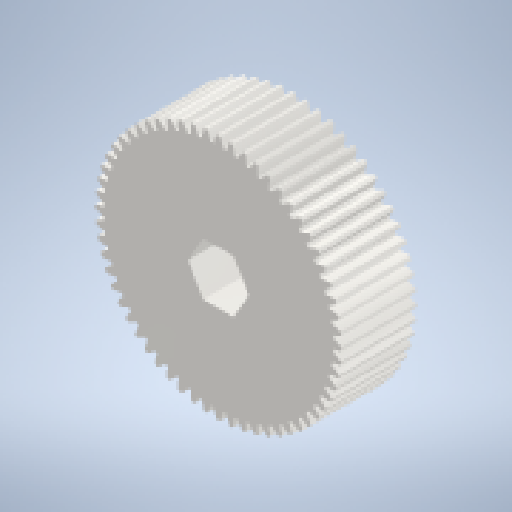
# Autodesk Inventor part: Spur Gear2
Saved by Autodesk Inventor 2024 (Build 280153020, 153B)
## iProperties
Created: 2024-04-17
Part Number: Spur Gear2
Material: Steel
Document SubType Name: Modeling
Designer: lvrectanus0
Categories: <?xml version="1.0" encoding="UTF-16"?> <MemberInstance><Categories><FamilyTemplate><FamilyTemplateParameter ValueType="xs:double" Id="1" ObjectReferenceKey="da_z" ObjectType="kUserParameterObject"/><FamilyTemplateParameter ValueType="xs:double" Id="2" ObjectReferenceKey="da_b" ObjectType="kUserParameterObject"/><FamilyTemplateParameter ValueType="xs:double" Id="3" ObjectReferenceKey="da_beta" ObjectType="kUserParameterObject"/><FamilyTemplateParameter ValueType="xs:double" Id="4" ObjectReferenceKey="da_da" ObjectType="kUserParameterObject"/><FamilyTemplateParameter ValueType="xs:double" Id="5" ObjectReferenceKey="da_aw" ObjectType="kUserParameterObject"/><FamilyTemplateParameter ValueType="xs:string" Id="6" ObjectReferenceKey="EAIAABAAAAC/AAAAAAAAAIAAAAAAAAAA" ObjectType="83910656" SubObjectId="SurfaceGeometry"/></FamilyTemplate><ParamToTemplateMap><ParamToTemplate CategoryParameter="//CategoryParameter[@InternalName='046C89C9-8512-4d59-83FE-43B91F4F132A']" TemplateParameter="1"/><ParamToTemplate CategoryParameter="//CategoryParameter[@InternalName='2552DF32-E462-4b46-AEBF-C6C7768E72AC']" TemplateParameter="2"/><ParamToTemplate CategoryParameter="//CategoryParameter[@InternalName='C9EE641D-15FC-4fae-A226-E94C4372FDD7']" TemplateParameter="3"/><ParamToTemplate><ParamToTemplate CategoryParameter="//CategoryParameter[@InternalName='00B6519A-459B-49c7-AD84-2E56D39A5744']" ConstantValue="0.000000"/></ParamToTemplate><ParamToTemplate><ParamToTemplate CategoryParameter="//CategoryParameter[@InternalName='04B31F0E-C7A6-4894-AA32-9629BEFACF47']" ConstantValue="1.000000"/></ParamToTemplate><ParamToTemplate><ParamToTemplate CategoryParameter="//CategoryParameter[@InternalName='43CBEC2E-7847-49e7-A936-2F7889FCB2D9']" ConstantValue="0.250000"/></ParamToTemplate><ParamToTemplate><ParamToTemplate CategoryParameter="//CategoryParameter[@InternalName='B1EFC894-105D-4ebd-86BF-FA20ED196853']" ConstantValue="0.350000"/></ParamToTemplate><ParamToTemplate><ParamToTemplate CategoryParameter="//CategoryParameter[@InternalName='51175063-3D10-4879-93E8-6246FE8B403D']" ConstantValue="2061532430.657340"/></ParamToTemplate><ParamToTemplate><ParamToTemplate CategoryParameter="//CategoryParameter[@InternalName='A3A52E27-4454-46a9-B0BD-C932399B70AF']" ConstantValue="0.300000"/></ParamToTemplate><ParamToTemplate><ParamToTemplate CategoryParameter="//CategoryParameter[@InternalName='91B76062-C214-41d9-B1B9-14D2AB99603D']" ConstantValue="0.079375"/></ParamToTemplate><ParamToTemplate><ParamToTemplate CategoryParameter="//CategoryParameter[@InternalName='374E806E-8B8A-4dda-A9AA-1039D6500AD2']" ConstantValue="12.598425"/></ParamToTemplate><ParamToTemplate><ParamToTemplate CategoryParameter="//CategoryParameter[@InternalName='2D373A89-B862-43d6-8D0B-0CBF12AB9F6C']" ConstantValue="0.349066"/></ParamToTemplate><ParamToTemplate CategoryParameter="//CategoryParameter[@InternalName='37777632-D6A2-4fac-9D53-DB8ACD95C989']" TemplateParameter="4"/><ParamToTemplate CategoryParameter="//CategoryParameter[@InternalName='FD1017F1-B727-4f7e-9707-0F86F1FF9423']" TemplateParameter="5"/><ParamToTemplate><ParamToTemplate CategoryParameter="//CategoryParameter[@InternalName='9E1B4470-B2D3-4ff1-B813-535BB4CDF51A']" ConstantValue="3523220.976809"/></ParamToTemplate><ParamToTemplate><ParamToTemplate CategoryParameter="//CategoryParameter[@InternalName='F8452263-BFF6-458c-9FB1-07C4B99E95CD']" ConstantValue="11397033.805607"/></ParamToTemplate><ParamToTemplate><ParamToTemplate CategoryParameter="//CategoryParameter[@InternalName='3E3BB259-FD49-497f-8171-6EBC954A3479']" ConstantValue="2.000000"/></ParamToTemplate><ParamToTemplate CategoryParameter="//CategoryParameter[@InternalName='27C3BAF2-7550-4e4b-AE2C-0DB134B7D9B7']" TemplateParameter="6"/></ParamToTemplateMap><Category DisplayName="Gear" InternalName="DC85795E-93AB-48d5-8EEE-5A27447B64BD" Mnemonic="Gear"><CategoryParameter DisplayName="z" InternalName="046C89C9-8512-4d59-83FE-43B91F4F132A" Mnemonic="z"/><CategoryParameter DisplayName="b" InternalName="2552DF32-E462-4b46-AEBF-C6C7768E72AC" Mnemonic="b"/><CategoryParameter DisplayName="||b|" InternalName="C9EE641D-15FC-4fae-A226-E94C4372FDD7" Mnemonic="beta"/><CategoryParameter DisplayName="x" InternalName="00B6519A-459B-49c7-AD84-2E56D39A5744" Mnemonic="x"/><CategoryParameter DisplayName="a*" InternalName="04B31F0E-C7A6-4894-AA32-9629BEFACF47" Mnemonic="a"/><CategoryParameter DisplayName="c*" InternalName="43CBEC2E-7847-49e7-A936-2F7889FCB2D9" Mnemonic="c"/><CategoryParameter DisplayName="r|.f|*" InternalName="B1EFC894-105D-4ebd-86BF-FA20ED196853" Mnemonic="rf"/><CategoryParameter DisplayName="E" InternalName="51175063-3D10-4879-93E8-6246FE8B403D" Mnemonic="E"/><CategoryParameter DisplayName="||m|" InternalName="A3A52E27-4454-46a9-B0BD-C932399B70AF" Mnemonic="mi"/><Category DisplayName="SpurGear" InternalName="26C5A22E-A91E-4dfd-A3B3-23CCAFAE1764" Mnemonic="SpurGear"><CategoryParameter DisplayName="m" InternalName="91B76062-C214-41d9-B1B9-14D2AB99603D" Mnemonic="m"/><CategoryParameter DisplayName="P" InternalName="374E806E-8B8A-4dda-A9AA-1039D6500AD2" Mnemonic="PP"/><CategoryParameter DisplayName="||a|" InternalName="2D373A89-B862-43d6-8D0B-0CBF12AB9F6C" Mnemonic="alpha"/><CategoryParameter DisplayName="d|.a|" InternalName="37777632-D6A2-4fac-9D53-DB8ACD95C989" Mnemonic="da"/><CategoryParameter DisplayName="a|.w|" InternalName="FD1017F1-B727-4f7e-9707-0F86F1FF9423" Mnemonic="aw"/><CategoryParameter DisplayName="||s||.Flim|" InternalName="9E1B4470-B2D3-4ff1-B813-535BB4CDF51A" Mnemonic="sFlim"/><CategoryParameter DisplayName="||s||.Hlim|" InternalName="F8452263-BFF6-458c-9FB1-07C4B99E95CD" Mnemonic="sHlim"/><CategoryParameter DisplayName="type" InternalName="3E3BB259-FD49-497f-8171-6EBC954A3479" Mnemonic="type"/><CategoryParameter DisplayName="PitchDiameter" InternalName="27C3BAF2-7550-4e4b-AE2C-0DB134B7D9B7" Mnemonic="IDS_PITCHDIAM"/></Category></Category></Categories></MemberInstance>
Density: 1 g/cm^3
Appearance: Steel
CustomPartVersion: 1
Author: lvrectanus0
Autodesk Inventor part; units mm, degrees
ref_plane "YZ Plane" through (0, 0, 0) normal (1, 0, 0) x (0, 1, 0)
ref_plane "XZ Plane" through (0, 0, 0) normal (0, 1, 0) x (-1, 0, 0)
ref_plane "XY Plane" through (0, 0, 0) normal (0, 0, 1) x (1, 0, 0)
sketch "Sketch1" plane through (0, 0, 0) normal (0, 0, 1) x (1, 0, 0)
  circle A0 centre (0, 0) radius 24.6062
  dimension "d0" = 49.2125
  constraints: 1 centre point
  measures "d0" diameter of A0
extrude "Extrusion1" add sketch "Sketch1" along normal blind 15
sketch "Sketch2" plane through (0, 0, 0) normal (0, 0, -1) x (-1, 0, 0)
  circle A0 centre (0, 0) radius 24.6062 projected
  circle A1 centre (0, 0) radius 23.8125
  dimension "d3" = 47.625
  constraints: 1 centre point, 1 coincident
  measures "d3" diameter of A1
surface extrude "Pitch Diameter" sketch "Sketch2" against normal through all shown no curves A1
ref_plane "Work Plane1" through (0, 0, 0) normal (1, 0, 0) x (0, 1, 0)
ref_plane "Work Plane2" through (0, 0, 0) normal (0.9986295, 0.052336, 0) x (0, 0, 1)
ref_plane "Work Plane3" through (0, 0, 7.5) normal (0, 0, -1) x (-1, 0, 0)
spur gear teeth "Spur Gear" teeth 60 pitch diameter 47.625 tip diameter 49.2125 root diameter 45.6406 face width 50.8 start plane through (0, 0, 0) normal (0, 0, -1) x (-1, 0, 0)
sketch "Sketch3" plane through (0, 0, 15) normal (0, 0, 1) x (1, 0, 0)
  line L0 (-3.0383, 5.2625) -> (3.0383, 5.2625)
  line L1 (3.0383, 5.2625) -> (6.0766, 0)
  line L2 (6.0766, 0) -> (3.0383, -5.2625)
  line L3 (3.0383, -5.2625) -> (-3.0383, -5.2625)
  line L4 (-3.0383, -5.2625) -> (-6.0766, 0)
  line L5 (-6.0766, 0) -> (-3.0383, 5.2625)
  line L6 (-3.0383, 5.2625) -> (3.0383, -5.2625)
  line L7 (-6.0766, 0) -> (6.0766, 0)
  line L8 (3.0383, 5.2625) -> (-3.0383, -5.2625)
  arc A0 (-2.8922, 24.4357) -> (-3.2745, 22.5842) centre (6.6821, 21.4931) ccw projected
  arc A1 (-3.2745, 22.5842) -> (-3.8646, 22.4907) centre (0, 0) ccw projected
  arc A2 (-3.8646, 22.4907) -> (-4.8004, 24.1334) centre (-12.9968, 18.3763) ccw projected
  arc A3 (-4.8004, 24.1334) -> (-5.4305, 23.9995) centre (0, 0) ccw projected
  arc A4 (-5.4305, 23.9995) -> (-5.6173, 22.1182) centre (4.3989, 22.0738) ccw projected
  arc A5 (-5.6173, 22.1182) -> (-6.1944, 21.9635) centre (0, 0) ccw projected
  arc A6 (-6.1944, 21.9635) -> (-7.2968, 23.4995) centre (-14.8464, 16.9171) ccw projected
  arc A7 (-7.2968, 23.4995) -> (-7.9094, 23.3004) centre (0, 0) ccw projected
  arc A8 (-7.9094, 23.3004) -> (-7.8985, 21.4098) centre (2.0674, 22.4127) ccw projected
  arc A9 (-7.8985, 21.4098) -> (-8.4562, 21.1957) centre (0, 0) ccw projected
  arc A10 (-8.4562, 21.1957) -> (-9.7132, 22.608) centre (-16.5334, 15.2725) ccw projected
  arc A11 (-9.7132, 22.608) -> (-10.3016, 22.346) centre (0, 0) ccw projected
  arc A12 (-10.3016, 22.346) -> (-10.0932, 20.4669) centre (-0.2867, 22.506) ccw projected
  arc A13 (-10.0932, 20.4669) -> (-10.6255, 20.1957) centre (0, 0) ccw projected
  arc A14 (-10.6255, 20.1957) -> (-12.0231, 21.4689) centre (-18.0393, 13.4606) ccw projected
  arc A15 (-12.0231, 21.4689) -> (-12.581, 21.1468) centre (0, 0) ccw projected
  arc A16 (-12.581, 21.1468) -> (-12.1773, 19.2998) centre (-2.6376, 22.3528) ccw projected
  arc A17 (-12.1773, 19.2998) -> (-12.6783, 18.9744) centre (0, 0) ccw projected
  arc A18 (-12.6783, 18.9744) -> (-14.2014, 20.0945) centre (-19.3475, 11.5013) ccw projected
  arc A19 (-14.2014, 20.0945) -> (-14.7225, 19.7159) centre (0, 0) ccw projected
  arc A20 (-14.7225, 19.7159) -> (-14.1279, 17.9212) centre (-4.9597, 21.9546) ccw projected
  arc A21 (-14.1279, 17.9212) -> (-14.5922, 17.5452) centre (0, 0) ccw projected
  arc A22 (-14.5922, 17.5452) -> (-16.224, 18.5) centre (-20.4437, 9.4159) ccw projected
  arc A23 (-16.224, 18.5) -> (-16.7027, 18.0689) centre (0, 0) ccw projected
  arc A24 (-16.7027, 18.0689) -> (-15.9238, 16.3462) centre (-7.2274, 21.3159) ccw projected
  arc A25 (-15.9238, 16.3462) -> (-16.3462, 15.9238) centre (0, 0) ccw projected
  arc A26 (-16.3462, 15.9238) -> (-18.0689, 16.7027) centre (-21.3159, 7.2274) ccw projected
  arc A27 (-18.0689, 16.7027) -> (-18.5, 16.224) centre (0, 0) ccw projected
  arc A28 (-18.5, 16.224) -> (-17.5452, 14.5922) centre (-9.4159, 20.4437) ccw projected
  arc A29 (-17.5452, 14.5922) -> (-17.9212, 14.1279) centre (0, 0) ccw projected
  arc A30 (-17.9212, 14.1279) -> (-19.7159, 14.7225) centre (-21.9546, 4.9597) ccw projected
  arc A31 (-19.7159, 14.7225) -> (-20.0945, 14.2014) centre (0, 0) ccw projected
  arc A32 (-20.0945, 14.2014) -> (-18.9744, 12.6783) centre (-11.5013, 19.3475) ccw projected
  arc A33 (-18.9744, 12.6783) -> (-19.2998, 12.1773) centre (0, 0) ccw projected
  arc A34 (-19.2998, 12.1773) -> (-21.1468, 12.581) centre (-22.3528, 2.6376) ccw projected
  arc A35 (-21.1468, 12.581) -> (-21.4689, 12.0231) centre (0, 0) ccw projected
  arc A36 (-21.4689, 12.0231) -> (-20.1957, 10.6255) centre (-13.4606, 18.0393) ccw projected
  arc A37 (-20.1957, 10.6255) -> (-20.4669, 10.0932) centre (0, 0) ccw projected
  arc A38 (-20.4669, 10.0932) -> (-22.346, 10.3016) centre (-22.506, 0.2867) ccw projected
  arc A39 (-22.346, 10.3016) -> (-22.608, 9.7132) centre (0, 0) ccw projected
  arc A40 (-22.608, 9.7132) -> (-21.1957, 8.4562) centre (-15.2725, 16.5334) ccw projected
  arc A41 (-21.1957, 8.4562) -> (-21.4098, 7.8985) centre (0, 0) ccw projected
  arc A42 (-21.4098, 7.8985) -> (-23.3004, 7.9094) centre (-22.4127, -2.0674) ccw projected
  arc A43 (-23.3004, 7.9094) -> (-23.4995, 7.2968) centre (0, 0) ccw projected
  arc A44 (-23.4995, 7.2968) -> (-21.9635, 6.1944) centre (-16.9171, 14.8464) ccw projected
  arc A45 (-21.9635, 6.1944) -> (-22.1182, 5.6173) centre (0, 0) ccw projected
  arc A46 (-22.1182, 5.6173) -> (-23.9995, 5.4305) centre (-22.0738, -4.3989) ccw projected
  arc A47 (-23.9995, 5.4305) -> (-24.1334, 4.8004) centre (0, 0) ccw projected
  arc A48 (-24.1334, 4.8004) -> (-22.4907, 3.8646) centre (-18.3763, 12.9968) ccw projected
  arc A49 (-22.4907, 3.8646) -> (-22.5842, 3.2745) centre (0, 0) ccw projected
  arc A50 (-22.5842, 3.2745) -> (-24.4357, 2.8922) centre (-21.4931, -6.6821) ccw projected
  arc A51 (-24.4357, 2.8922) -> (-24.503, 2.2515) centre (0, 0) ccw projected
  arc A52 (-24.503, 2.2515) -> (-22.7715, 1.4925) centre (-19.6341, 11.0048) ccw projected
  arc A53 (-22.7715, 1.4925) -> (-22.8027, 0.8959) centre (0, 0) ccw projected
  arc A54 (-22.8027, 0.8959) -> (-24.6041, 0.3221) centre (-20.6769, -8.8921) ccw projected
  arc A55 (-24.6041, 0.3221) -> (-24.6041, -0.3221) centre (0, 0) ccw projected
  arc A56 (-24.6041, -0.3221) -> (-22.8027, -0.8959) centre (-20.6769, 8.8921) ccw projected
  arc A57 (-22.8027, -0.8959) -> (-22.7715, -1.4925) centre (0, 0) ccw projected
  arc A58 (-22.7715, -1.4925) -> (-24.503, -2.2515) centre (-19.6341, -11.0048) ccw projected
  arc A59 (-24.503, -2.2515) -> (-24.4357, -2.8922) centre (0, 0) ccw projected
  arc A60 (-24.4357, -2.8922) -> (-22.5842, -3.2745) centre (-21.4931, 6.6821) ccw projected
  arc A61 (-22.5842, -3.2745) -> (-22.4907, -3.8646) centre (0, 0) ccw projected
  arc A62 (-22.4907, -3.8646) -> (-24.1334, -4.8004) centre (-18.3763, -12.9968) ccw projected
  arc A63 (-24.1334, -4.8004) -> (-23.9995, -5.4305) centre (0, 0) ccw projected
  arc A64 (-23.9995, -5.4305) -> (-22.1182, -5.6173) centre (-22.0738, 4.3989) ccw projected
  arc A65 (-22.1182, -5.6173) -> (-21.9635, -6.1944) centre (0, 0) ccw projected
  arc A66 (-21.9635, -6.1944) -> (-23.4995, -7.2968) centre (-16.9171, -14.8464) ccw projected
  arc A67 (-23.4995, -7.2968) -> (-23.3004, -7.9094) centre (0, 0) ccw projected
  arc A68 (-23.3004, -7.9094) -> (-21.4098, -7.8985) centre (-22.4127, 2.0674) ccw projected
  arc A69 (-21.4098, -7.8985) -> (-21.1957, -8.4562) centre (0, 0) ccw projected
  arc A70 (-21.1957, -8.4562) -> (-22.608, -9.7132) centre (-15.2725, -16.5334) ccw projected
  arc A71 (-22.608, -9.7132) -> (-22.346, -10.3016) centre (0, 0) ccw projected
  arc A72 (-22.346, -10.3016) -> (-20.4669, -10.0932) centre (-22.506, -0.2867) ccw projected
  arc A73 (-20.4669, -10.0932) -> (-20.1957, -10.6255) centre (0, 0) ccw projected
  arc A74 (-20.1957, -10.6255) -> (-21.4689, -12.0231) centre (-13.4606, -18.0393) ccw projected
  arc A75 (-21.4689, -12.0231) -> (-21.1468, -12.581) centre (0, 0) ccw projected
  arc A76 (-21.1468, -12.581) -> (-19.2998, -12.1773) centre (-22.3528, -2.6376) ccw projected
  arc A77 (-19.2998, -12.1773) -> (-18.9744, -12.6783) centre (0, 0) ccw projected
  arc A78 (-18.9744, -12.6783) -> (-20.0945, -14.2014) centre (-11.5013, -19.3475) ccw projected
  arc A79 (-20.0945, -14.2014) -> (-19.7159, -14.7225) centre (0, 0) ccw projected
  arc A80 (-19.7159, -14.7225) -> (-17.9212, -14.1279) centre (-21.9546, -4.9597) ccw projected
  arc A81 (-17.9212, -14.1279) -> (-17.5452, -14.5922) centre (0, 0) ccw projected
  arc A82 (-17.5452, -14.5922) -> (-18.5, -16.224) centre (-9.4159, -20.4437) ccw projected
  arc A83 (-18.5, -16.224) -> (-18.0689, -16.7027) centre (0, 0) ccw projected
  arc A84 (-18.0689, -16.7027) -> (-16.3462, -15.9238) centre (-21.3159, -7.2274) ccw projected
  arc A85 (-16.3462, -15.9238) -> (-15.9238, -16.3462) centre (0, 0) ccw projected
  arc A86 (-15.9238, -16.3462) -> (-16.7027, -18.0689) centre (-7.2274, -21.3159) ccw projected
  arc A87 (-16.7027, -18.0689) -> (-16.224, -18.5) centre (0, 0) ccw projected
  arc A88 (-16.224, -18.5) -> (-14.5922, -17.5452) centre (-20.4437, -9.4159) ccw projected
  arc A89 (-14.5922, -17.5452) -> (-14.1279, -17.9212) centre (0, 0) ccw projected
  arc A90 (-14.1279, -17.9212) -> (-14.7225, -19.7159) centre (-4.9597, -21.9546) ccw projected
  arc A91 (-14.7225, -19.7159) -> (-14.2014, -20.0945) centre (0, 0) ccw projected
  arc A92 (-14.2014, -20.0945) -> (-12.6783, -18.9744) centre (-19.3475, -11.5013) ccw projected
  arc A93 (-12.6783, -18.9744) -> (-12.1773, -19.2998) centre (0, 0) ccw projected
  arc A94 (-12.1773, -19.2998) -> (-12.581, -21.1468) centre (-2.6376, -22.3528) ccw projected
  arc A95 (-12.581, -21.1468) -> (-12.0231, -21.4689) centre (0, 0) ccw projected
  arc A96 (-12.0231, -21.4689) -> (-10.6255, -20.1957) centre (-18.0393, -13.4606) ccw projected
  arc A97 (-10.6255, -20.1957) -> (-10.0932, -20.4669) centre (0, 0) ccw projected
  arc A98 (-10.0932, -20.4669) -> (-10.3016, -22.346) centre (-0.2867, -22.506) ccw projected
  arc A99 (-10.3016, -22.346) -> (-9.7132, -22.608) centre (0, 0) ccw projected
  arc A100 (-9.7132, -22.608) -> (-8.4562, -21.1957) centre (-16.5334, -15.2725) ccw projected
  arc A101 (-8.4562, -21.1957) -> (-7.8985, -21.4098) centre (0, 0) ccw projected
  arc A102 (-7.8985, -21.4098) -> (-7.9094, -23.3004) centre (2.0674, -22.4127) ccw projected
  arc A103 (-7.9094, -23.3004) -> (-7.2968, -23.4995) centre (0, 0) ccw projected
  arc A104 (-7.2968, -23.4995) -> (-6.1944, -21.9635) centre (-14.8464, -16.9171) ccw projected
  arc A105 (-6.1944, -21.9635) -> (-5.6173, -22.1182) centre (0, 0) ccw projected
  arc A106 (-5.6173, -22.1182) -> (-5.4305, -23.9995) centre (4.3989, -22.0738) ccw projected
  arc A107 (-5.4305, -23.9995) -> (-4.8004, -24.1334) centre (0, 0) ccw projected
  arc A108 (-4.8004, -24.1334) -> (-3.8646, -22.4907) centre (-12.9968, -18.3763) ccw projected
  arc A109 (-3.8646, -22.4907) -> (-3.2745, -22.5842) centre (0, 0) ccw projected
  arc A110 (-3.2745, -22.5842) -> (-2.8922, -24.4357) centre (6.6821, -21.4931) ccw projected
  arc A111 (-2.8922, -24.4357) -> (-2.2515, -24.503) centre (0, 0) ccw projected
  arc A112 (-2.2515, -24.503) -> (-1.4925, -22.7715) centre (-11.0048, -19.6341) ccw projected
  arc A113 (-1.4925, -22.7715) -> (-0.8959, -22.8027) centre (0, 0) ccw projected
  arc A114 (-0.8959, -22.8027) -> (-0.3221, -24.6041) centre (8.8921, -20.6769) ccw projected
  arc A115 (-0.3221, -24.6041) -> (0.3221, -24.6041) centre (0, 0) ccw projected
  arc A116 (0.3221, -24.6041) -> (0.8959, -22.8027) centre (-8.8921, -20.6769) ccw projected
  arc A117 (0.8959, -22.8027) -> (1.4925, -22.7715) centre (0, 0) ccw projected
  arc A118 (1.4925, -22.7715) -> (2.2515, -24.503) centre (11.0048, -19.6341) ccw projected
  arc A119 (2.2515, -24.503) -> (2.8922, -24.4357) centre (0, 0) ccw projected
  arc A120 (2.8922, -24.4357) -> (3.2745, -22.5842) centre (-6.6821, -21.4931) ccw projected
  arc A121 (3.2745, -22.5842) -> (3.8646, -22.4907) centre (0, 0) ccw projected
  arc A122 (3.8646, -22.4907) -> (4.8004, -24.1334) centre (12.9968, -18.3763) ccw projected
  arc A123 (4.8004, -24.1334) -> (5.4305, -23.9995) centre (0, 0) ccw projected
  arc A124 (5.4305, -23.9995) -> (5.6173, -22.1182) centre (-4.3989, -22.0738) ccw projected
  arc A125 (5.6173, -22.1182) -> (6.1944, -21.9635) centre (0, 0) ccw projected
  arc A126 (6.1944, -21.9635) -> (7.2968, -23.4995) centre (14.8464, -16.9171) ccw projected
  arc A127 (7.2968, -23.4995) -> (7.9094, -23.3004) centre (0, 0) ccw projected
  arc A128 (7.9094, -23.3004) -> (7.8985, -21.4098) centre (-2.0674, -22.4127) ccw projected
  arc A129 (7.8985, -21.4098) -> (8.4562, -21.1957) centre (0, 0) ccw projected
  arc A130 (8.4562, -21.1957) -> (9.7132, -22.608) centre (16.5334, -15.2725) ccw projected
  arc A131 (9.7132, -22.608) -> (10.3016, -22.346) centre (0, 0) ccw projected
  arc A132 (10.3016, -22.346) -> (10.0932, -20.4669) centre (0.2867, -22.506) ccw projected
  arc A133 (10.0932, -20.4669) -> (10.6255, -20.1957) centre (0, 0) ccw projected
  arc A134 (10.6255, -20.1957) -> (12.0231, -21.4689) centre (18.0393, -13.4606) ccw projected
  arc A135 (12.0231, -21.4689) -> (12.581, -21.1468) centre (0, 0) ccw projected
  arc A136 (12.581, -21.1468) -> (12.1773, -19.2998) centre (2.6376, -22.3528) ccw projected
  arc A137 (12.1773, -19.2998) -> (12.6783, -18.9744) centre (0, 0) ccw projected
  arc A138 (12.6783, -18.9744) -> (14.2014, -20.0945) centre (19.3475, -11.5013) ccw projected
  arc A139 (14.2014, -20.0945) -> (14.7225, -19.7159) centre (0, 0) ccw projected
  arc A140 (14.7225, -19.7159) -> (14.1279, -17.9212) centre (4.9597, -21.9546) ccw projected
  arc A141 (14.1279, -17.9212) -> (14.5922, -17.5452) centre (0, 0) ccw projected
  arc A142 (14.5922, -17.5452) -> (16.224, -18.5) centre (20.4437, -9.4159) ccw projected
  arc A143 (16.224, -18.5) -> (16.7027, -18.0689) centre (0, 0) ccw projected
  arc A144 (16.7027, -18.0689) -> (15.9238, -16.3462) centre (7.2274, -21.3159) ccw projected
  arc A145 (15.9238, -16.3462) -> (16.3462, -15.9238) centre (0, 0) ccw projected
  arc A146 (16.3462, -15.9238) -> (18.0689, -16.7027) centre (21.3159, -7.2274) ccw projected
  arc A147 (18.0689, -16.7027) -> (18.5, -16.224) centre (0, 0) ccw projected
  arc A148 (18.5, -16.224) -> (17.5452, -14.5922) centre (9.4159, -20.4437) ccw projected
  arc A149 (17.5452, -14.5922) -> (17.9212, -14.1279) centre (0, 0) ccw projected
  arc A150 (17.9212, -14.1279) -> (19.7159, -14.7225) centre (21.9546, -4.9597) ccw projected
  arc A151 (19.7159, -14.7225) -> (20.0945, -14.2014) centre (0, 0) ccw projected
  arc A152 (20.0945, -14.2014) -> (18.9744, -12.6783) centre (11.5013, -19.3475) ccw projected
  arc A153 (18.9744, -12.6783) -> (19.2998, -12.1773) centre (0, 0) ccw projected
  arc A154 (19.2998, -12.1773) -> (21.1468, -12.581) centre (22.3528, -2.6376) ccw projected
  arc A155 (21.1468, -12.581) -> (21.4689, -12.0231) centre (0, 0) ccw projected
  arc A156 (21.4689, -12.0231) -> (20.1957, -10.6255) centre (13.4606, -18.0393) ccw projected
  arc A157 (20.1957, -10.6255) -> (20.4669, -10.0932) centre (0, 0) ccw projected
  arc A158 (20.4669, -10.0932) -> (22.346, -10.3016) centre (22.506, -0.2867) ccw projected
  arc A159 (22.346, -10.3016) -> (22.608, -9.7132) centre (0, 0) ccw projected
  arc A160 (22.608, -9.7132) -> (21.1957, -8.4562) centre (15.2725, -16.5334) ccw projected
  arc A161 (21.1957, -8.4562) -> (21.4098, -7.8985) centre (0, 0) ccw projected
  arc A162 (21.4098, -7.8985) -> (23.3004, -7.9094) centre (22.4127, 2.0674) ccw projected
  arc A163 (23.3004, -7.9094) -> (23.4995, -7.2968) centre (0, 0) ccw projected
  arc A164 (23.4995, -7.2968) -> (21.9635, -6.1944) centre (16.9171, -14.8464) ccw projected
  arc A165 (21.9635, -6.1944) -> (22.1182, -5.6173) centre (0, 0) ccw projected
  arc A166 (22.1182, -5.6173) -> (23.9995, -5.4305) centre (22.0738, 4.3989) ccw projected
  arc A167 (23.9995, -5.4305) -> (24.1334, -4.8004) centre (0, 0) ccw projected
  arc A168 (24.1334, -4.8004) -> (22.4907, -3.8646) centre (18.3763, -12.9968) ccw projected
  arc A169 (22.4907, -3.8646) -> (22.5842, -3.2745) centre (0, 0) ccw projected
  arc A170 (22.5842, -3.2745) -> (24.4357, -2.8922) centre (21.4931, 6.6821) ccw projected
  arc A171 (24.4357, -2.8922) -> (24.503, -2.2515) centre (0, 0) ccw projected
  arc A172 (24.503, -2.2515) -> (22.7715, -1.4925) centre (19.6341, -11.0048) ccw projected
  arc A173 (22.7715, -1.4925) -> (22.8027, -0.8959) centre (0, 0) ccw projected
  arc A174 (22.8027, -0.8959) -> (24.6041, -0.3221) centre (20.6769, 8.8921) ccw projected
  arc A175 (24.6041, -0.3221) -> (24.6041, 0.3221) centre (0, 0) ccw projected
  arc A176 (24.6041, 0.3221) -> (22.8027, 0.8959) centre (20.6769, -8.8921) ccw projected
  arc A177 (22.8027, 0.8959) -> (22.7715, 1.4925) centre (0, 0) ccw projected
  arc A178 (22.7715, 1.4925) -> (24.503, 2.2515) centre (19.6341, 11.0048) ccw projected
  arc A179 (24.503, 2.2515) -> (24.4357, 2.8922) centre (0, 0) ccw projected
  arc A180 (24.4357, 2.8922) -> (22.5842, 3.2745) centre (21.4931, -6.6821) ccw projected
  arc A181 (22.5842, 3.2745) -> (22.4907, 3.8646) centre (0, 0) ccw projected
  arc A182 (22.4907, 3.8646) -> (24.1334, 4.8004) centre (18.3763, 12.9968) ccw projected
  arc A183 (24.1334, 4.8004) -> (23.9995, 5.4305) centre (0, 0) ccw projected
  arc A184 (23.9995, 5.4305) -> (22.1182, 5.6173) centre (22.0738, -4.3989) ccw projected
  arc A185 (22.1182, 5.6173) -> (21.9635, 6.1944) centre (0, 0) ccw projected
  arc A186 (21.9635, 6.1944) -> (23.4995, 7.2968) centre (16.9171, 14.8464) ccw projected
  arc A187 (23.4995, 7.2968) -> (23.3004, 7.9094) centre (0, 0) ccw projected
  arc A188 (23.3004, 7.9094) -> (21.4098, 7.8985) centre (22.4127, -2.0674) ccw projected
  arc A189 (21.4098, 7.8985) -> (21.1957, 8.4562) centre (0, 0) ccw projected
  arc A190 (21.1957, 8.4562) -> (22.608, 9.7132) centre (15.2725, 16.5334) ccw projected
  arc A191 (22.608, 9.7132) -> (22.346, 10.3016) centre (0, 0) ccw projected
  arc A192 (22.346, 10.3016) -> (20.4669, 10.0932) centre (22.506, 0.2867) ccw projected
  arc A193 (20.4669, 10.0932) -> (20.1957, 10.6255) centre (0, 0) ccw projected
  arc A194 (20.1957, 10.6255) -> (21.4689, 12.0231) centre (13.4606, 18.0393) ccw projected
  arc A195 (21.4689, 12.0231) -> (21.1468, 12.581) centre (0, 0) ccw projected
  arc A196 (21.1468, 12.581) -> (19.2998, 12.1773) centre (22.3528, 2.6376) ccw projected
  arc A197 (19.2998, 12.1773) -> (18.9744, 12.6783) centre (0, 0) ccw projected
  arc A198 (18.9744, 12.6783) -> (20.0945, 14.2014) centre (11.5013, 19.3475) ccw projected
  arc A199 (20.0945, 14.2014) -> (19.7159, 14.7225) centre (0, 0) ccw projected
  arc A200 (19.7159, 14.7225) -> (17.9212, 14.1279) centre (21.9546, 4.9597) ccw projected
  arc A201 (17.9212, 14.1279) -> (17.5452, 14.5922) centre (0, 0) ccw projected
  arc A202 (17.5452, 14.5922) -> (18.5, 16.224) centre (9.4159, 20.4437) ccw projected
  arc A203 (18.5, 16.224) -> (18.0689, 16.7027) centre (0, 0) ccw projected
  arc A204 (18.0689, 16.7027) -> (16.3462, 15.9238) centre (21.3159, 7.2274) ccw projected
  arc A205 (16.3462, 15.9238) -> (15.9238, 16.3462) centre (0, 0) ccw projected
  arc A206 (15.9238, 16.3462) -> (16.7027, 18.0689) centre (7.2274, 21.3159) ccw projected
  arc A207 (16.7027, 18.0689) -> (16.224, 18.5) centre (0, 0) ccw projected
  arc A208 (16.224, 18.5) -> (14.5922, 17.5452) centre (20.4437, 9.4159) ccw projected
  arc A209 (14.5922, 17.5452) -> (14.1279, 17.9212) centre (0, 0) ccw projected
  arc A210 (14.1279, 17.9212) -> (14.7225, 19.7159) centre (4.9597, 21.9546) ccw projected
  arc A211 (14.7225, 19.7159) -> (14.2014, 20.0945) centre (0, 0) ccw projected
  arc A212 (14.2014, 20.0945) -> (12.6783, 18.9744) centre (19.3475, 11.5013) ccw projected
  arc A213 (12.6783, 18.9744) -> (12.1773, 19.2998) centre (0, 0) ccw projected
  arc A214 (12.1773, 19.2998) -> (12.581, 21.1468) centre (2.6376, 22.3528) ccw projected
  arc A215 (12.581, 21.1468) -> (12.0231, 21.4689) centre (0, 0) ccw projected
  arc A216 (12.0231, 21.4689) -> (10.6255, 20.1957) centre (18.0393, 13.4606) ccw projected
  arc A217 (10.6255, 20.1957) -> (10.0932, 20.4669) centre (0, 0) ccw projected
  arc A218 (10.0932, 20.4669) -> (10.3016, 22.346) centre (0.2867, 22.506) ccw projected
  arc A219 (10.3016, 22.346) -> (9.7132, 22.608) centre (0, 0) ccw projected
  arc A220 (9.7132, 22.608) -> (8.4562, 21.1957) centre (16.5334, 15.2725) ccw projected
  arc A221 (8.4562, 21.1957) -> (7.8985, 21.4098) centre (0, 0) ccw projected
  arc A222 (7.8985, 21.4098) -> (7.9094, 23.3004) centre (-2.0674, 22.4127) ccw projected
  arc A223 (7.9094, 23.3004) -> (7.2968, 23.4995) centre (0, 0) ccw projected
  arc A224 (7.2968, 23.4995) -> (6.1944, 21.9635) centre (14.8464, 16.9171) ccw projected
  arc A225 (6.1944, 21.9635) -> (5.6173, 22.1182) centre (0, 0) ccw projected
  arc A226 (5.6173, 22.1182) -> (5.4305, 23.9995) centre (-4.3989, 22.0738) ccw projected
  arc A227 (5.4305, 23.9995) -> (4.8004, 24.1334) centre (0, 0) ccw projected
  arc A228 (4.8004, 24.1334) -> (3.8646, 22.4907) centre (12.9968, 18.3763) ccw projected
  arc A229 (3.8646, 22.4907) -> (3.2745, 22.5842) centre (0, 0) ccw projected
  arc A230 (3.2745, 22.5842) -> (2.8922, 24.4357) centre (-6.6821, 21.4931) ccw projected
  arc A231 (2.8922, 24.4357) -> (2.2515, 24.503) centre (0, 0) ccw projected
  arc A232 (2.2515, 24.503) -> (1.4925, 22.7715) centre (11.0048, 19.6341) ccw projected
  arc A233 (1.4925, 22.7715) -> (0.8959, 22.8027) centre (0, 0) ccw projected
  arc A234 (0.8959, 22.8027) -> (0.3221, 24.6041) centre (-8.8921, 20.6769) ccw projected
  arc A235 (0.3221, 24.6041) -> (-0.3221, 24.6041) centre (0, 0) ccw projected
  arc A236 (-0.3221, 24.6041) -> (-0.8959, 22.8027) centre (8.8921, 20.6769) ccw projected
  arc A237 (-0.8959, 22.8027) -> (-1.4925, 22.7715) centre (0, 0) ccw projected
  arc A238 (-1.4925, 22.7715) -> (-2.2515, 24.503) centre (-11.0048, 19.6341) ccw projected
  arc A239 (-2.2515, 24.503) -> (-2.8922, 24.4357) centre (0, 0) ccw projected
  dimension "d21" = 10.525
  dimension "d22" = 10.525
  dimension "d23" = 10.525
  constraints: 18 end point, 3 equal length, 1 coincident, 1 horizontal, 1 midpoint, 1 parallel
  measures "d21" distance between parallel lines of L3 L0
  measures "d22" distance between parallel lines of L4 L1
  measures "d23" distance between parallel lines of L2 L5
extrude "Extrusion2" cut sketch "Sketch3" against normal through all contours L6 L7 L5 | L0 L8 L6 | L1 L7 L8 | L7 L8 L4 | L7 L2 L6 | L6 L3 L8
equation "\"d0\" = da_da"
equation "\"d3\" = da_d"
equation "\"d15\" = da_aw"
equation "\"d19\" = da_aw"
equation "\"da_da\" = 49.2125"
equation "\"da_d\" = 47.625"
equation "\"da_aw\" = 28.575"
body "Solid1"
body "Srf1"
